Autodesk Fusion 360 part; units mm, degrees
(part 2 of 3)
sketch "Skizze16" plane through (0, 0, 3) normal (0, 0, -1) x (1, 0, 0)
  circle A0 centre (16.9122, 11.6198) radius 1
  circle A1 centre (77.0127, 20.2056) radius 2.5
  line L0 (81.1827, 15.7656) -> (79.9827, 16.6656)
  arc A2 (81.2427, 18.3456) -> (79.9827, 16.6656) centre (80.6127, 17.5056) ccw
  line L1 (81.2427, 18.3456) -> (82.4427, 17.4456)
  arc A3 (81.1827, 15.7656) -> (82.4427, 17.4456) centre (81.8127, 16.6056) ccw
  line L2 (72.7827, 22.0656) -> (71.5827, 22.9656)
  arc A4 (72.8427, 24.6456) -> (71.5827, 22.9656) centre (72.2127, 23.8056) ccw
  line L3 (72.8427, 24.6456) -> (74.0427, 23.7456)
  arc A5 (72.7827, 22.0656) -> (74.0427, 23.7456) centre (73.4127, 22.9056) ccw
  line L4 (72.5727, 16.0356) -> (73.4727, 17.2356)
  arc A6 (75.1527, 15.9756) -> (73.4727, 17.2356) centre (74.3127, 16.6056) ccw
  line L5 (75.1527, 15.9756) -> (74.2527, 14.7756)
  arc A7 (72.5727, 16.0356) -> (74.2527, 14.7756) centre (73.4127, 15.4056) ccw
  arc A8 (82.9846, 19.6249) -> (82.5459, 22.526) centre (77.0127, 20.2056) ccw
  arc A9 (83.8074, 23.8534) -> (82.5459, 22.526) centre (83.4681, 22.9127) ccw
  line L6 (83.8074, 23.8534) -> (87.1568, 22.6453)
  arc A10 (87.4261, 20.9112) -> (87.1568, 22.6453) centre (86.8175, 21.7046) ccw
  line L7 (87.4261, 20.9112) -> (84.5885, 18.7346)
  arc A11 (82.9846, 19.6249) -> (84.5885, 18.7346) centre (83.9799, 19.5281) ccw
  arc A12 (81.4527, 24.3756) -> (79.7727, 25.6356) centre (80.6127, 25.0056) ccw
  line L8 (81.4527, 24.3756) -> (80.5527, 23.1756)
  arc A13 (78.8727, 24.4356) -> (80.5527, 23.1756) centre (79.7127, 23.8056) ccw
  line L9 (78.8727, 24.4356) -> (79.7727, 25.6356)
  circle A14 centre (7.0127, 10.2056) radius 1
  line L10 (60.0865, 20.8143) -> (43.481, 18.4383)
  arc A15 (25.7008, 16.7003) -> (43.481, 18.4383) centre (15.1527, 216.4219) ccw
  line L11 (25.7008, 16.7003) -> (-2.9873, 15.1851)
  line L12 (-2.9873, 15.1851) -> (-2.9873, 11.7056)
  line L13 (-2.9873, 11.7056) -> (2.0127, 11.7056)
  arc A16 (2.0127, 8.7056) -> (2.0127, 11.7056) centre (2.0127, 10.2056) ccw
  line L14 (2.0127, 8.7056) -> (-2.9873, 8.7056)
  line L15 (-2.9873, 8.7056) -> (-2.9873, 5.7056)
  line L16 (-2.9873, 5.7056) -> (9.5815, 5.7056)
  arc A17 (9.5815, 5.7056) -> (14.161, 6.237) centre (9.5815, 25.7056) ccw
  line L17 (14.161, 6.237) -> (31.1237, 10.2271)
  arc A18 (39.9015, 11.8821) -> (31.1237, 10.2271) centre (54.0216, -87.116) ccw
  line L18 (39.9015, 11.8821) -> (60.934, 14.8819)
  arc A19 (72.34, 13.1475) -> (60.934, 14.8819) centre (63.758, -4.9177) ccw
  arc A20 (72.34, 13.1475) -> (74.5856, 13.1978) centre (73.4127, 15.4056) ccw
  arc A21 (77.8619, 14.266) -> (74.5856, 13.1978) centre (79.2772, 4.3667) ccw
  arc A22 (81.3049, 14.1577) -> (77.8619, 14.266) centre (79.2738, 4.3662) ccw
  arc A23 (81.3049, 14.1577) -> (83.2245, 14.5424) centre (81.8127, 16.6056) ccw
  line L19 (83.2245, 14.5424) -> (91.9997, 20.5467)
  arc A24 (91.9997, 20.5467) -> (91.4886, 24.0993) centre (90.8703, 22.1973) ccw
  line L20 (91.4886, 24.0993) -> (81.3855, 27.3832)
  arc A25 (81.3855, 27.3832) -> (79.4398, 27.2134) centre (80.6127, 25.0056) ccw
  arc A26 (76.1636, 26.1452) -> (79.4398, 27.2134) centre (74.7483, 36.0446) ccw
  arc A27 (72.7205, 26.2535) -> (76.1636, 26.1452) centre (74.7517, 36.045) ccw
  arc A28 (72.7205, 26.2535) -> (70.5506, 25.6731) centre (72.2127, 23.8056) ccw
  arc A29 (60.0865, 20.8143) -> (70.5506, 25.6731) centre (57.2537, 40.6127) ccw
  circle A30 centre (16.9122, 11.6198) radius 1.5
  circle A31 centre (7.0127, 10.2056) radius 1.5
  dimension "d177" = 3
  dimension "d178" = 3
  constraint concentric A0 A30
  constraint concentric A14 A31
  measures "d177" diameter of A30
  measures "d178" diameter of A31
extrude "Extrusion1'''" cut sketch "Skizze16" against normal blind 3 contours A30 | A31 sketch seen with x (-0.6, -0.8, 0) y (0.8, -0.6, 0) z (0, 0, 1) at (-23.2665, 43.7378, -3) bodies 10 in component "Component''"
sketch "Skizze17" plane through (0, 0, 3) normal (0, 0, -1) x (1, 0, 0)
  circle A0 centre (-22.8868, 11.6198) radius 1
  circle A1 centre (-82.9873, 20.2056) radius 2.5
  line L0 (-85.9573, 16.6656) -> (-87.1573, 15.7656)
  arc A2 (-88.4173, 17.4456) -> (-87.1573, 15.7656) centre (-87.7873, 16.6056) ccw
  line L1 (-88.4173, 17.4456) -> (-87.2173, 18.3456)
  arc A3 (-85.9573, 16.6656) -> (-87.2173, 18.3456) centre (-86.5873, 17.5056) ccw
  line L2 (-77.5573, 22.9656) -> (-78.7573, 22.0656)
  arc A4 (-80.0173, 23.7456) -> (-78.7573, 22.0656) centre (-79.3873, 22.9056) ccw
  line L3 (-80.0173, 23.7456) -> (-78.8173, 24.6456)
  arc A5 (-77.5573, 22.9656) -> (-78.8173, 24.6456) centre (-78.1873, 23.8056) ccw
  line L4 (-79.4473, 17.2356) -> (-78.5473, 16.0356)
  arc A6 (-80.2273, 14.7756) -> (-78.5473, 16.0356) centre (-79.3873, 15.4056) ccw
  line L5 (-80.2273, 14.7756) -> (-81.1273, 15.9756)
  arc A7 (-79.4473, 17.2356) -> (-81.1273, 15.9756) centre (-80.2873, 16.6056) ccw
  arc A8 (-88.5204, 22.526) -> (-88.9591, 19.6249) centre (-82.9873, 20.2056) ccw
  arc A9 (-90.563, 18.7346) -> (-88.9591, 19.6249) centre (-89.9544, 19.5281) ccw
  line L6 (-90.563, 18.7346) -> (-93.4007, 20.9112)
  arc A10 (-93.1314, 22.6453) -> (-93.4007, 20.9112) centre (-92.7921, 21.7046) ccw
  line L7 (-93.1314, 22.6453) -> (-89.7819, 23.8534)
  arc A11 (-88.5204, 22.526) -> (-89.7819, 23.8534) centre (-89.4426, 22.9127) ccw
  arc A12 (-85.7473, 25.6356) -> (-87.4273, 24.3756) centre (-86.5873, 25.0056) ccw
  line L8 (-85.7473, 25.6356) -> (-84.8473, 24.4356)
  arc A13 (-86.5273, 23.1756) -> (-84.8473, 24.4356) centre (-85.6873, 23.8056) ccw
  line L9 (-86.5273, 23.1756) -> (-87.4273, 24.3756)
  circle A14 centre (-12.9873, 10.2056) radius 1
  line L10 (-49.4555, 18.4383) -> (-66.061, 20.8143)
  arc A15 (-76.5252, 25.6731) -> (-66.061, 20.8143) centre (-63.2282, 40.6127) ccw
  arc A16 (-76.5252, 25.6731) -> (-78.6951, 26.2535) centre (-78.1873, 23.8056) ccw
  arc A17 (-82.1381, 26.1452) -> (-78.6951, 26.2535) centre (-80.7262, 36.045) ccw
  arc A18 (-85.4144, 27.2134) -> (-82.1381, 26.1452) centre (-80.7228, 36.0446) ccw
  arc A19 (-85.4144, 27.2134) -> (-87.3601, 27.3832) centre (-86.5873, 25.0056) ccw
  line L11 (-87.3601, 27.3832) -> (-97.4631, 24.0993)
  arc A20 (-97.4631, 24.0993) -> (-97.9743, 20.5467) centre (-96.8449, 22.1973) ccw
  line L12 (-97.9743, 20.5467) -> (-89.199, 14.5424)
  arc A21 (-89.199, 14.5424) -> (-87.2795, 14.1577) centre (-87.7873, 16.6056) ccw
  arc A22 (-83.8364, 14.266) -> (-87.2795, 14.1577) centre (-85.2483, 4.3662) ccw
  arc A23 (-80.5602, 13.1978) -> (-83.8364, 14.266) centre (-85.2517, 4.3667) ccw
  arc A24 (-80.5602, 13.1978) -> (-78.3145, 13.1475) centre (-79.3873, 15.4056) ccw
  arc A25 (-66.9085, 14.8819) -> (-78.3145, 13.1475) centre (-69.7326, -4.9177) ccw
  line L13 (-66.9085, 14.8819) -> (-45.8761, 11.8821)
  arc A26 (-37.0983, 10.2271) -> (-45.8761, 11.8821) centre (-59.9962, -87.116) ccw
  line L14 (-37.0983, 10.2271) -> (-20.1356, 6.237)
  arc A27 (-20.1356, 6.237) -> (-15.556, 5.7056) centre (-15.556, 25.7056) ccw
  line L15 (-15.556, 5.7056) -> (-2.9873, 5.7056)
  line L16 (-2.9873, 5.7056) -> (-2.9873, 8.7056)
  line L17 (-2.9873, 8.7056) -> (-7.9873, 8.7056)
  arc A28 (-7.9873, 11.7056) -> (-7.9873, 8.7056) centre (-7.9873, 10.2056) ccw
  line L18 (-7.9873, 11.7056) -> (-2.9873, 11.7056)
  line L19 (-2.9873, 11.7056) -> (-2.9873, 15.1851)
  line L20 (-2.9873, 15.1851) -> (-31.6754, 16.7003)
  arc A29 (-49.4555, 18.4383) -> (-31.6754, 16.7003) centre (-21.1273, 216.4219) ccw
  circle A30 centre (-22.8868, 11.6198) radius 1.5
  circle A31 centre (-12.9873, 10.2056) radius 1.5
  dimension "d181" = 3
  dimension "d182" = 3
  constraint concentric A0 A30
  constraint concentric A14 A31
  measures "d181" diameter of A30
  measures "d182" diameter of A31
extrude "Extrusion1''''" cut sketch "Skizze17" against normal blind 3 contours A30 | A31 sketch seen with x (0.6, 0.8, 0) y (0.8, -0.6, 0) z (0, 0, -1) at (-18.7221, 22.2947, 6) bodies 11 in component "Component'''"
sketch "Skizze18" plane through (0, 0, 3) normal (0, 0, -1) x (1, 0, 0)
  circle A0 centre (-20.7786, -30.2009) radius 1
  arc A1 (-65.0305, -85.2371) -> (-65.3296, -83.1585) centre (-65.18, -84.1978) ccw
  line L0 (-65.0305, -85.2371) -> (-66.5152, -85.4508)
  arc A2 (-66.8143, -83.3722) -> (-66.5152, -85.4508) centre (-66.6647, -84.4115) ccw
  line L1 (-66.8143, -83.3722) -> (-65.3296, -83.1585)
  arc A3 (-65.3866, -87.3355) -> (-67.1533, -87.8235) centre (-66.1634, -87.9652) ccw
  arc A4 (-65.3866, -87.3355) -> (-63.0387, -89.0932) centre (-60.7259, -83.5569) ccw
  arc A5 (-63.0094, -90.9259) -> (-63.0387, -89.0932) centre (-63.4241, -90.016) ccw
  line L2 (-63.0094, -90.9259) -> (-66.2541, -92.4046)
  arc A6 (-67.6587, -91.3529) -> (-66.2541, -92.4046) centre (-66.6688, -91.4947) ccw
  line L3 (-67.6587, -91.3529) -> (-67.1533, -87.8235)
  arc A7 (-60.5412, -77.4685) -> (-62.6198, -77.7676) centre (-61.5805, -77.6181) ccw
  line L4 (-60.5412, -77.4685) -> (-60.3275, -78.9532)
  arc A8 (-62.4061, -79.2523) -> (-60.3275, -78.9532) centre (-61.3668, -79.1028) ccw
  line L5 (-62.4061, -79.2523) -> (-62.6198, -77.7676)
  circle A9 centre (-60.7259, -83.5569) radius 2.5
  circle A10 centre (-12.9873, -19.7944) radius 1
  arc A11 (-59.0457, -87.8615) -> (-61.1243, -88.1606) centre (-60.085, -88.011) ccw
  line L6 (-59.0457, -87.8615) -> (-58.832, -89.3462)
  arc A12 (-60.9106, -89.6453) -> (-58.832, -89.3462) centre (-59.8713, -89.4957) ccw
  line L7 (-60.9106, -89.6453) -> (-61.1243, -88.1606)
  line L8 (-56.4213, -81.8767) -> (-54.9366, -81.663)
  arc A13 (-54.6375, -83.7416) -> (-54.9366, -81.663) centre (-54.7871, -82.7023) ccw
  line L9 (-54.6375, -83.7416) -> (-56.1222, -83.9553)
  arc A14 (-56.4213, -81.8767) -> (-56.1222, -83.9553) centre (-56.2718, -82.916) ccw
  arc A15 (-68.3484, -81.9285) -> (-69.636, -83.9975) centre (-66.6647, -84.4115) ccw
  line L10 (-69.636, -83.9975) -> (-71.0974, -94.488)
  arc A16 (-71.0974, -94.488) -> (-68.294, -96.587) centre (-69.1165, -94.7639) ccw
  line L11 (-68.294, -96.587) -> (-58.6376, -92.2303)
  arc A17 (-58.6376, -92.2303) -> (-57.0144, -90.411) centre (-59.8713, -89.4957) ccw
  arc A18 (-53.1034, -85.1853) -> (-57.0144, -90.411) centre (-47.4911, -93.4619) ccw
  arc A19 (-53.1034, -85.1853) -> (-51.788, -82.7784) centre (-54.7871, -82.7023) ccw
  arc A20 (-47.8066, -71.3016) -> (-51.788, -82.7784) centre (-31.7945, -83.2854) ccw
  line L12 (-47.8066, -71.3016) -> (-30.9597, -48.7917)
  arc A21 (-25.5822, -42.2094) -> (-30.9597, -48.7917) centre (49.1009, -108.7108) ccw
  line L13 (-25.5822, -42.2094) -> (-21.1501, -37.232)
  arc A22 (-21.1501, -37.232) -> (-16.2298, -30.7009) centre (-58.4917, -3.9813) ccw
  line L14 (-16.2298, -30.7009) -> (-13.6512, -26.6224)
  arc A23 (-9.4251, -24.2944) -> (-13.6512, -26.6224) centre (-9.4251, -29.2944) ccw
  line L15 (-9.4251, -24.2944) -> (-2.9873, -24.2944)
  line L16 (-2.9873, -24.2944) -> (-2.9873, -21.2944)
  line L17 (-2.9873, -21.2944) -> (-7.9873, -21.2944)
  arc A24 (-7.9873, -18.2944) -> (-7.9873, -21.2944) centre (-7.9873, -19.7944) ccw
  line L18 (-7.9873, -18.2944) -> (-2.9873, -18.2944)
  line L19 (-2.9873, -18.2944) -> (-2.9873, -15.2944)
  line L20 (-2.9873, -15.2944) -> (-13.8886, -15.2944)
  arc A25 (-13.8886, -15.2944) -> (-18.1306, -17.6477) centre (-13.8886, -20.2944) ccw
  line L21 (-18.1306, -17.6477) -> (-30.9484, -38.1918)
  arc A26 (-35.7499, -45.2053) -> (-30.9484, -38.1918) centre (-115.7896, 14.7418) ccw
  line L22 (-35.7499, -45.2053) -> (-52.6043, -67.7088)
  arc A27 (-62.4977, -74.7617) -> (-52.6043, -67.7088) centre (-68.6122, -55.7193) ccw
  arc A28 (-62.4977, -74.7617) -> (-64.4374, -76.7028) centre (-61.5805, -77.6181) ccw
  arc A29 (-68.3484, -81.9285) -> (-64.4374, -76.7028) centre (-73.9607, -73.6518) ccw
  circle A30 centre (-20.7786, -30.2009) radius 1.5
  circle A31 centre (-12.9873, -19.7944) radius 1.5
  dimension "d185" = 3
  dimension "d186" = 3
  constraint concentric A0 A30
  constraint concentric A10 A31
  measures "d185" diameter of A30
  measures "d186" diameter of A31
extrude "Extrusion1'''''" cut sketch "Skizze18" against normal blind 3 contours A30 | A31 sketch seen with x (0.989831, -0.142249, 0) y (-0.142249, -0.989831, 0) z (0, 0, -1) at (-24.4554, -5.7072, 6) bodies 12 in component "Component''''"
sketch "Skizze19" plane through (0, 0, 0) normal (0, 0, -1) x (1, 0, 0)
  circle A0 centre (-10.9873, -60.7944) radius 1
  circle A1 centre (7.0127, -49.2944) radius 1
  circle A2 centre (-10.9873, -12.7944) radius 1
  circle A3 centre (-22.8868, 11.6198) radius 1
  circle A4 centre (7.0127, -19.7944) radius 1
  circle A5 centre (7.0127, 10.2056) radius 1
  arc A6 (4.4716, -52.3625) -> (3.467, -47.3835) centre (-2.4249, -51.1632) ccw
  line L0 (4.4716, -52.3625) -> (3.9295, -55.4797)
  arc A7 (-0.0113, -58.7944) -> (3.9295, -55.4797) centre (-0.0113, -54.7944) ccw
  line L1 (-0.0113, -58.7944) -> (-5.9632, -58.7944)
  arc A8 (-9.904, -55.4797) -> (-5.9632, -58.7944) centre (-5.9632, -54.7944) ccw
  line L2 (-9.904, -55.4797) -> (-10.4462, -52.3625)
  arc A9 (-9.4415, -47.3835) -> (-10.4462, -52.3625) centre (-3.5497, -51.1632) ccw
  line L3 (-9.4415, -47.3835) -> (-4.0198, -38.932)
  arc A10 (-3.1781, -38.4719) -> (-4.0198, -38.932) centre (-3.1781, -39.4719) ccw
  line L4 (-3.1781, -38.4719) -> (-2.7964, -38.4719)
  arc A11 (-1.9547, -38.932) -> (-2.7964, -38.4719) centre (-2.7964, -39.4719) ccw
  line L5 (-1.9547, -38.932) -> (3.467, -47.3835)
  arc A12 (-10.6956, -31.3597) -> (-10.9873, -32.7585) centre (-7.4873, -32.7585) ccw
  arc A13 (-10.6956, -31.3597) -> (-10.4873, -30.3606) centre (-12.9873, -30.3606) ccw
  line L6 (-10.4873, -30.3606) -> (-10.4873, -28.821)
  arc A14 (-8.6429, -28.2852) -> (-10.4873, -28.821) centre (-9.4873, -28.821) ccw
  line L7 (-8.6429, -28.2852) -> (-6.2521, -32.0531)
  arc A15 (-5.9408, -33.1247) -> (-6.2521, -32.0531) centre (-7.9408, -33.1247) ccw
  line L8 (-5.9408, -33.1247) -> (-5.9408, -35.784)
  arc A16 (-6.2574, -36.8639) -> (-5.9408, -35.784) centre (-7.9408, -35.784) ccw
  line L9 (-6.2574, -36.8639) -> (-9.1456, -41.3661)
  arc A17 (-10.9873, -40.8261) -> (-9.1456, -41.3661) centre (-9.9873, -40.8261) ccw
  line L10 (-10.9873, -40.8261) -> (-10.9873, -32.7585)
  circle A18 centre (5.0127, -12.7944) radius 1
  arc A19 (-2.8219, -30.4719) -> (-1.9776, -30.0077) centre (-2.8219, -29.4719) ccw
  line L11 (-2.8219, -30.4719) -> (-3.1526, -30.4719)
  arc A20 (-3.997, -30.0077) -> (-3.1526, -30.4719) centre (-3.1526, -29.4719) ccw
  line L12 (-3.997, -30.0077) -> (-6.6478, -25.8302)
  arc A21 (-5.8034, -24.2944) -> (-6.6478, -25.8302) centre (-5.8034, -25.2944) ccw
  line L13 (-5.8034, -24.2944) -> (-0.1711, -24.2944)
  arc A22 (0.6732, -25.8302) -> (-0.1711, -24.2944) centre (-0.1711, -25.2944) ccw
  line L14 (0.6732, -25.8302) -> (-1.9776, -30.0077)
  line L15 (2.0127, 8.7056) -> (-7.9873, 8.7056)
  arc A23 (-7.9873, 11.7056) -> (-7.9873, 8.7056) centre (-7.9873, 10.2056) ccw
  line L16 (-7.9873, 11.7056) -> (2.0127, 11.7056)
  arc A24 (2.0127, 8.7056) -> (2.0127, 11.7056) centre (2.0127, 10.2056) ccw
  circle A25 centre (16.9122, 11.6198) radius 1
  circle A26 centre (14.804, -30.2009) radius 1
  circle A27 centre (-12.9873, 10.2056) radius 1
  circle A28 centre (-12.9873, -19.7944) radius 1
  circle A29 centre (5.0127, 3.2056) radius 1
  line L17 (2.0127, -21.2944) -> (-7.9873, -21.2944)
  arc A30 (-7.9873, -18.2944) -> (-7.9873, -21.2944) centre (-7.9873, -19.7944) ccw
  line L18 (-7.9873, -18.2944) -> (2.0127, -18.2944)
  arc A31 (2.0127, -21.2944) -> (2.0127, -18.2944) centre (2.0127, -19.7944) ccw
  circle A32 centre (5.0127, -60.7944) radius 1
  circle A33 centre (-12.9873, -49.2944) radius 1
  circle A34 centre (-10.9873, 3.2056) radius 1
  circle A35 centre (-20.7786, -30.2009) radius 1
  line L19 (3.5127, -1.2944) -> (3.5127, -8.2944)
  arc A36 (0.5127, -11.2944) -> (3.5127, -8.2944) centre (0.5127, -8.2944) ccw
  line L20 (0.5127, -11.2944) -> (-6.4873, -11.2944)
  arc A37 (-9.4873, -8.2944) -> (-6.4873, -11.2944) centre (-6.4873, -8.2944) ccw
  line L21 (-9.4873, -8.2944) -> (-9.4873, -1.2944)
  arc A38 (-6.4873, 1.7056) -> (-9.4873, -1.2944) centre (-6.4873, -1.2944) ccw
  line L22 (-6.4873, 1.7056) -> (0.5127, 1.7056)
  arc A39 (3.5127, -1.2944) -> (0.5127, 1.7056) centre (0.5127, -1.2944) ccw
  arc A40 (4.5127, -28.821) -> (2.6684, -28.2852) centre (3.5127, -28.821) ccw
  line L23 (4.5127, -28.821) -> (4.5127, -30.3606)
  arc A41 (4.5127, -30.3606) -> (4.7211, -31.3597) centre (7.0127, -30.3606) ccw
  arc A42 (5.0127, -32.7585) -> (4.7211, -31.3597) centre (1.5127, -32.7585) ccw
  line L24 (5.0127, -32.7585) -> (5.0127, -40.8261)
  arc A43 (3.171, -41.3661) -> (5.0127, -40.8261) centre (4.0127, -40.8261) ccw
  line L25 (3.171, -41.3661) -> (0.2829, -36.8639)
  arc A44 (-0.0338, -35.784) -> (0.2829, -36.8639) centre (1.9662, -35.784) ccw
  line L26 (-0.0338, -35.784) -> (-0.0338, -33.1247)
  arc A45 (0.2775, -32.0531) -> (-0.0338, -33.1247) centre (1.9662, -33.1247) ccw
  line L27 (0.2775, -32.0531) -> (2.6684, -28.2852)
  circle A46 centre (-12.9873, -29.2944) radius 1
  circle A47 centre (7.0127, -29.2944) radius 1
  arc A48 (8.5127, -45.5527) -> (9.1794, -48.0472) centre (13.5127, -45.5527) ccw
  line L28 (8.5127, -45.5527) -> (8.5127, -33.6896)
  arc A49 (11.133, -32.6921) -> (8.5127, -33.6896) centre (10.0127, -33.6896) ccw
  line L29 (11.133, -32.6921) -> (11.5192, -33.1258)
  arc A50 (11.5192, -33.1258) -> (18.5356, -27.8727) centre (14.804, -30.2009) ccw
  line L30 (18.5356, -27.8727) -> (12.3422, -17.946)
  arc A51 (10.8263, -12.6526) -> (12.3422, -17.946) centre (20.8263, -12.6526) ccw
  line L31 (10.8263, -12.6526) -> (10.8263, 1.4922)
  arc A52 (14.6814, 6.3594) -> (10.8263, 1.4922) centre (15.8263, 1.4922) ccw
  line L32 (14.6814, 6.3594) -> (17.9678, 7.1324)
  arc A53 (17.9678, 7.1324) -> (16.6691, 16.2233) centre (16.9122, 11.6198) ccw
  line L33 (16.6691, 16.2233) -> (-0.3502, 15.3244)
  arc A54 (-5.6243, 15.3244) -> (-0.3502, 15.3244) centre (-2.9873, 65.2548) ccw
  line L34 (-5.6243, 15.3244) -> (-22.6436, 16.2233)
  arc A55 (-22.6436, 16.2233) -> (-23.9423, 7.1324) centre (-22.8868, 11.6198) ccw
  line L35 (-23.9423, 7.1324) -> (-20.6559, 6.3594)
  arc A56 (-16.8008, 1.4922) -> (-20.6559, 6.3594) centre (-21.8008, 1.4922) ccw
  line L36 (-16.8008, 1.4922) -> (-16.8008, -12.6526)
  arc A57 (-18.3167, -17.946) -> (-16.8008, -12.6526) centre (-26.8008, -12.6526) ccw
  line L37 (-18.3167, -17.946) -> (-24.5102, -27.8727)
  arc A58 (-24.5102, -27.8727) -> (-17.4938, -33.1258) centre (-20.7786, -30.2009) ccw
  line L38 (-17.4938, -33.1258) -> (-17.1075, -32.6921)
  arc A59 (-14.4873, -33.6896) -> (-17.1075, -32.6921) centre (-15.9873, -33.6896) ccw
  line L39 (-14.4873, -33.6896) -> (-14.4873, -45.5527)
  arc A60 (-15.1539, -48.0472) -> (-14.4873, -45.5527) centre (-19.4873, -45.5527) ccw
  arc A61 (-15.1539, -48.0472) -> (-14.9651, -50.8235) centre (-12.9873, -49.2944) ccw
  arc A62 (-14.0092, -52.946) -> (-14.9651, -50.8235) centre (-18.9209, -53.8816) ccw
  line L40 (-14.0092, -52.946) -> (-13.1609, -57.3995)
  arc A63 (-13.349, -59.9746) -> (-13.1609, -57.3995) centre (-18.0726, -58.335) ccw
  arc A64 (-13.349, -59.9746) -> (-10.0897, -63.1277) centre (-10.9873, -60.7944) ccw
  arc A65 (-8.2947, -62.7944) -> (-10.0897, -63.1277) centre (-8.2947, -67.7944) ccw
  line L41 (-8.2947, -62.7944) -> (2.3201, -62.7944)
  arc A66 (4.1152, -63.1277) -> (2.3201, -62.7944) centre (2.3201, -67.7944) ccw
  arc A67 (4.1152, -63.1277) -> (7.3745, -59.9746) centre (5.0127, -60.7944) ccw
  arc A68 (7.1863, -57.3995) -> (7.3745, -59.9746) centre (12.098, -58.335) ccw
  line L42 (7.1863, -57.3995) -> (8.0346, -52.946)
  arc A69 (8.9906, -50.8235) -> (8.0346, -52.946) centre (12.9463, -53.8816) ccw
  arc A70 (8.9906, -50.8235) -> (9.1794, -48.0472) centre (7.0127, -49.2944) ccw
  circle A71 centre (-22.8868, 11.6198) radius 1.5
  circle A72 centre (-12.9873, 10.2056) radius 1.5
  circle A73 centre (7.0127, 10.2056) radius 1.5
  circle A74 centre (16.9122, 11.6198) radius 1.5
  circle A75 centre (7.0127, -19.7944) radius 1.5
  circle A76 centre (-12.9873, -19.7944) radius 1.5
  circle A77 centre (-20.7786, -30.2009) radius 1.5
  circle A78 centre (-12.9873, -29.2944) radius 1.5
  circle A79 centre (7.0127, -29.2944) radius 1.5
  circle A80 centre (14.804, -30.2009) radius 1.5
  circle A81 centre (-12.9873, -49.2944) radius 1.5
  circle A82 centre (-10.9873, -60.7944) radius 1.5
  circle A83 centre (5.0127, -60.7944) radius 1.5
  circle A84 centre (7.0127, -49.2944) radius 1.5
  circle A85 centre (5.0127, -60.7944) radius 3.5
  circle A86 centre (-10.9873, -60.7944) radius 3.5
  circle A87 centre (-12.9873, -49.2944) radius 3.5
  circle A88 centre (7.0127, -49.2944) radius 3.5
  circle A89 centre (-12.9873, -29.2944) radius 3.5
  circle A90 centre (7.0127, -29.2944) radius 3.5
  circle A91 centre (-10.9873, 3.2056) radius 1.5
  circle A92 centre (-10.9873, -12.7944) radius 1.5
  circle A93 centre (5.0127, -12.7944) radius 1.5
  circle A94 centre (5.0127, 3.2056) radius 1.5
  dimension "d189" = 3
  dimension "d190" = 3
  dimension "d191" = 3
  dimension "d192" = 3
  dimension "d193" = 3
  dimension "d194" = 3
  dimension "d195" = 3
  dimension "d196" = 3
  dimension "d197" = 3
  dimension "d198" = 3
  dimension "d199" = 3
  dimension "d200" = 3
  dimension "d201" = 3
  dimension "d202" = 3
  dimension "d203" = 7
  dimension "d204" = 7
  dimension "d205" = 7
  dimension "d206" = 7
  dimension "d207" = 7
  dimension "d208" = 7
  dimension "d235" = 3
  dimension "d236" = 3
  dimension "d237" = 3
  dimension "d238" = 3
  constraint concentric A3 A71
  constraint concentric A27 A72
  constraint concentric A5 A73
  constraint concentric A25 A74
  constraint concentric A4 A75
  constraint concentric A28 A76
  constraint concentric A35 A77
  constraint concentric A46 A78
  constraint concentric A47 A79
  constraint concentric A26 A80
  constraint concentric A33 A81
  constraint concentric A0 A82
  constraint concentric A32 A83
  constraint concentric A1 A84
  constraint concentric A83 A85
  constraint concentric A82 A86
  constraint concentric A33 A87
  constraint concentric A84 A88
  constraint concentric A78 A89
  constraint concentric A79 A90
  constraint concentric A34 A91
  constraint concentric A2 A92
  constraint concentric A18 A93
  constraint concentric A29 A94
  measures "d189" diameter of A71
  measures "d190" diameter of A72
  measures "d191" diameter of A73
  measures "d192" diameter of A74
  measures "d193" diameter of A75
  measures "d194" diameter of A76
  measures "d195" diameter of A77
  measures "d196" diameter of A78
  measures "d197" diameter of A79
  measures "d198" diameter of A80
  measures "d199" diameter of A81
  measures "d200" diameter of A82
  measures "d201" diameter of A83
  measures "d202" diameter of A84
  measures "d203" diameter of A85
  measures "d204" diameter of A86
  measures "d205" diameter of A87
  measures "d206" diameter of A88
  measures "d207" diameter of A89
  measures "d208" diameter of A90
  measures "d235" diameter of A91
  measures "d236" diameter of A92
  measures "d237" diameter of A93
  measures "d238" diameter of A94
extrude "Extrusion1''''''" cut sketch "Skizze19" against normal blind 3 contours A71 | A72 | A73 | A74 | A75 | A76 | A77 | A80 | A82 | A83 | A91 | A92 | A93 | A94 sketch seen with x (1, 0, 0) y (0, 1, 0) z (0, 0, 1) at (2.9873, 0.2056, 0) bodies 13 in component "Component'''''"
extrude "Extrusion2'''" add sketch "Skizze19" against normal blind 3 contours L41 A66 A67 A68 A85 | A63 A64 A65 L41 A86 picked at (7.6038, -59.5802) picked at (-13.5291, -59.4774) sketch seen with x (1, 0, 0) y (0, 1, 0) z (0, 0, 1) at (2.9873, 0.2056, 0) bodies 13 in component "Component'''''"
fillet "Abrundung1''" radius 5 4 edges at (-10.0971, 58.1978, 1.5) (-5.1277, 63, 1.5) (5.1277, 63, 1.5) (10.0971, 58.1978, 1.5) on bodies 13 in component "Component'''''"
sketch "Skizze20" plane through (0, 0, 3) normal (0, 0, 1) x (-1, 0, 0)
  circle A0 centre (12.9873, 10.2056) radius 1.5
  circle A1 centre (-14.804, -30.2009) radius 1.5
  circle A2 centre (10.9873, -60.7944) radius 1.5
  circle A3 centre (20.7786, -30.2009) radius 1.5
  circle A4 centre (-5.0127, -60.7944) radius 1.5
  circle A5 centre (-7.0127, -19.7944) radius 1.5
  circle A6 centre (-7.0127, 10.2056) radius 1.5
  circle A7 centre (22.8868, 11.6198) radius 1.5
  circle A8 centre (12.9873, -19.7944) radius 1.5
  circle A9 centre (-16.9122, 11.6198) radius 1.5
  line L0 (-3.467, -47.3835) -> (1.9547, -38.932)
  arc A10 (2.7964, -38.4719) -> (1.9547, -38.932) centre (2.7964, -39.4719) ccw
  line L1 (2.7964, -38.4719) -> (3.1781, -38.4719)
  arc A11 (4.0198, -38.932) -> (3.1781, -38.4719) centre (3.1781, -39.4719) ccw
  line L2 (4.0198, -38.932) -> (9.4415, -47.3835)
  line L3 (10.4462, -52.3625) -> (9.904, -55.4797)
  arc A12 (5.9632, -58.7944) -> (9.904, -55.4797) centre (5.9632, -54.7944) ccw
  line L4 (5.9632, -58.7944) -> (0.0113, -58.7944)
  arc A13 (-3.9295, -55.4797) -> (0.0113, -58.7944) centre (0.0113, -54.7944) ccw
  line L5 (-3.9295, -55.4797) -> (-4.4716, -52.3625)
  line L6 (10.9873, -32.7585) -> (10.9873, -40.8261)
  arc A14 (9.1456, -41.3661) -> (10.9873, -40.8261) centre (9.9873, -40.8261) ccw
  line L7 (9.1456, -41.3661) -> (6.2574, -36.8639)
  arc A15 (5.9408, -35.784) -> (6.2574, -36.8639) centre (7.9408, -35.784) ccw
  line L8 (5.9408, -35.784) -> (5.9408, -33.1247)
  arc A16 (6.2521, -32.0531) -> (5.9408, -33.1247) centre (7.9408, -33.1247) ccw
  line L9 (6.2521, -32.0531) -> (8.6429, -28.2852)
  arc A17 (1.9776, -30.0077) -> (2.8219, -30.4719) centre (2.8219, -29.4719) ccw
  line L10 (1.9776, -30.0077) -> (-0.6732, -25.8302)
  arc A18 (0.1711, -24.2944) -> (-0.6732, -25.8302) centre (0.1711, -25.2944) ccw
  line L11 (0.1711, -24.2944) -> (5.8034, -24.2944)
  arc A19 (6.6478, -25.8302) -> (5.8034, -24.2944) centre (5.8034, -25.2944) ccw
  line L12 (6.6478, -25.8302) -> (3.997, -30.0077)
  arc A20 (3.1526, -30.4719) -> (3.997, -30.0077) centre (3.1526, -29.4719) ccw
  line L13 (3.1526, -30.4719) -> (2.8219, -30.4719)
  line L14 (7.9873, 8.7056) -> (-2.0127, 8.7056)
  arc A21 (-2.0127, 11.7056) -> (-2.0127, 8.7056) centre (-2.0127, 10.2056) ccw
  line L15 (-2.0127, 11.7056) -> (7.9873, 11.7056)
  arc A22 (7.9873, 8.7056) -> (7.9873, 11.7056) centre (7.9873, 10.2056) ccw
  line L16 (7.9873, -21.2944) -> (-2.0127, -21.2944)
  arc A23 (-2.0127, -18.2944) -> (-2.0127, -21.2944) centre (-2.0127, -19.7944) ccw
  line L17 (-2.0127, -18.2944) -> (7.9873, -18.2944)
  arc A24 (7.9873, -21.2944) -> (7.9873, -18.2944) centre (7.9873, -19.7944) ccw
  line L18 (-3.5127, -8.2944) -> (-3.5127, -1.2944)
  arc A25 (-0.5127, 1.7056) -> (-3.5127, -1.2944) centre (-0.5127, -1.2944) ccw
  line L19 (-0.5127, 1.7056) -> (6.4873, 1.7056)
  arc A26 (9.4873, -1.2944) -> (6.4873, 1.7056) centre (6.4873, -1.2944) ccw
  line L20 (9.4873, -1.2944) -> (9.4873, -8.2944)
  arc A27 (6.4873, -11.2944) -> (9.4873, -8.2944) centre (6.4873, -8.2944) ccw
  line L21 (6.4873, -11.2944) -> (-0.5127, -11.2944)
  arc A28 (-3.5127, -8.2944) -> (-0.5127, -11.2944) centre (-0.5127, -8.2944) ccw
  line L22 (-2.6684, -28.2852) -> (-0.2775, -32.0531)
  arc A29 (0.0338, -33.1247) -> (-0.2775, -32.0531) centre (-1.9662, -33.1247) ccw
  line L23 (0.0338, -33.1247) -> (0.0338, -35.784)
  arc A30 (-0.2829, -36.8639) -> (0.0338, -35.784) centre (-1.9662, -35.784) ccw
  line L24 (-0.2829, -36.8639) -> (-3.171, -41.3661)
  arc A31 (-5.0127, -40.8261) -> (-3.171, -41.3661) centre (-4.0127, -40.8261) ccw
  line L25 (-5.0127, -40.8261) -> (-5.0127, -32.7585)
  line L26 (-8.0346, -52.946) -> (-7.5111, -55.6946)
  arc A32 (-8.0639, -59.0797) -> (-7.5111, -55.6946) centre (-12.4228, -56.6301) ccw
  arc A33 (-8.0639, -59.0797) -> (-3.0273, -63.6767) centre (-5.0127, -60.7944) ccw
  arc A34 (-0.1909, -62.7944) -> (-3.0273, -63.6767) centre (-0.1909, -67.7944) ccw
  line L27 (-0.1909, -62.7944) -> (6.1654, -62.7944)
  arc A35 (9.0018, -63.6767) -> (6.1654, -62.7944) centre (6.1654, -67.7944) ccw
  arc A36 (9.0018, -63.6767) -> (14.0385, -59.0797) centre (10.9873, -60.7944) ccw
  arc A37 (13.4856, -55.6946) -> (14.0385, -59.0797) centre (18.3973, -56.6301) ccw
  line L28 (13.4856, -55.6946) -> (14.0092, -52.946)
  line L29 (14.4873, -45.5527) -> (14.4873, -33.6896)
  arc A38 (17.1075, -32.6921) -> (14.4873, -33.6896) centre (15.9873, -33.6896) ccw
  line L30 (17.1075, -32.6921) -> (17.4938, -33.1258)
  arc A39 (17.4938, -33.1258) -> (24.5102, -27.8727) centre (20.7786, -30.2009) ccw
  line L31 (24.5102, -27.8727) -> (18.3167, -17.946)
  arc A40 (16.8008, -12.6526) -> (18.3167, -17.946) centre (26.8008, -12.6526) ccw
  line L32 (16.8008, -12.6526) -> (16.8008, 1.4922)
  arc A41 (20.6559, 6.3594) -> (16.8008, 1.4922) centre (21.8008, 1.4922) ccw
  line L33 (20.6559, 6.3594) -> (23.9423, 7.1324)
  arc A42 (23.9423, 7.1324) -> (22.6436, 16.2233) centre (22.8868, 11.6198) ccw
  line L34 (22.6436, 16.2233) -> (5.6243, 15.3244)
  arc A43 (0.3502, 15.3244) -> (5.6243, 15.3244) centre (2.9873, 65.2548) ccw
  line L35 (0.3502, 15.3244) -> (-16.6691, 16.2233)
  arc A44 (-16.6691, 16.2233) -> (-17.9678, 7.1324) centre (-16.9122, 11.6198) ccw
  line L36 (-17.9678, 7.1324) -> (-14.6814, 6.3594)
  arc A45 (-10.8263, 1.4922) -> (-14.6814, 6.3594) centre (-15.8263, 1.4922) ccw
  line L37 (-10.8263, 1.4922) -> (-10.8263, -12.6526)
  arc A46 (-12.3422, -17.946) -> (-10.8263, -12.6526) centre (-20.8263, -12.6526) ccw
  line L38 (-12.3422, -17.946) -> (-18.5356, -27.8727)
  arc A47 (-18.5356, -27.8727) -> (-11.5192, -33.1258) centre (-14.804, -30.2009) ccw
  line L39 (-11.5192, -33.1258) -> (-11.133, -32.6921)
  arc A48 (-8.5127, -33.6896) -> (-11.133, -32.6921) centre (-10.0127, -33.6896) ccw
  line L40 (-8.5127, -33.6896) -> (-8.5127, -45.5527)
  circle A49 centre (12.9873, -29.2944) radius 2
  circle A50 centre (-7.0127, -29.2944) radius 2
  circle A51 centre (-7.0127, -49.2944) radius 1
  circle A52 centre (12.9873, -49.2944) radius 1
  circle A53 centre (12.9873, -29.2944) radius 1
  circle A54 centre (-7.0127, -29.2944) radius 1
  arc A55 (-3.467, -47.3835) -> (-4.4716, -52.3625) centre (2.4249, -51.1632) ccw
  arc A56 (10.4462, -52.3625) -> (9.4415, -47.3835) centre (3.5497, -51.1632) ccw
  arc A57 (-9.1794, -48.0472) -> (-8.5127, -45.5527) centre (-13.5127, -45.5527) ccw
  arc A58 (-9.1794, -48.0472) -> (-8.9906, -50.8235) centre (-7.0127, -49.2944) ccw
  arc A59 (-8.0346, -52.946) -> (-8.9906, -50.8235) centre (-12.9463, -53.8816) ccw
  arc A60 (14.9651, -50.8235) -> (14.0092, -52.946) centre (18.9209, -53.8816) ccw
  arc A61 (14.9651, -50.8235) -> (15.1539, -48.0472) centre (12.9873, -49.2944) ccw
  arc A62 (14.4873, -45.5527) -> (15.1539, -48.0472) centre (19.4873, -45.5527) ccw
  arc A63 (10.9873, -32.7585) -> (10.6956, -31.3597) centre (7.4873, -32.7585) ccw
  arc A64 (-4.7211, -31.3597) -> (-5.0127, -32.7585) centre (-1.5127, -32.7585) ccw
  arc A65 (10.4873, -28.821) -> (8.6429, -28.2852) centre (9.4873, -28.821) ccw
  line L41 (10.4873, -28.821) -> (10.4873, -30.3606)
  arc A66 (10.4873, -30.3606) -> (10.6956, -31.3597) centre (12.9873, -30.3606) ccw
  arc A67 (-2.6684, -28.2852) -> (-4.5127, -28.821) centre (-3.5127, -28.821) ccw
  arc A68 (-4.7211, -31.3597) -> (-4.5127, -30.3606) centre (-7.0127, -30.3606) ccw
  line L42 (-4.5127, -30.3606) -> (-4.5127, -28.821)
  circle A69 centre (10.9873, -12.7944) radius 1.5
  circle A70 centre (10.9873, 3.2056) radius 1.5
  circle A71 centre (-5.0127, -12.7944) radius 1.5
  circle A72 centre (-5.0127, 3.2056) radius 1.5
  dimension "d217" = 4
  dimension "d218" = 4
  measures "d217" diameter of A49
  measures "d218" diameter of A50
extrude "Extrusion3'" cut sketch "Skizze20" along normal blind 7 contours A49 | A50 | A53 | A54 sketch seen with x (1, 0, 0) y (0, 1, 0) z (0, 0, 1) at (2.9873, 0.2056, -6) bodies 8 in component "Component"
extrude "Extrusion2''''" cut sketch "Skizze20" along normal blind 7 contours A49 | A50 | A53 | A54 sketch seen with x (0.989831, -0.142249, 0) y (-0.142249, -0.989831, 0) z (0, 0, -1) at (-24.4554, -5.7072, 6) bodies 12 in component "Component''''"
extrude "Extrusion1'''''''" cut sketch "Skizze20" along normal blind 7 contours A49 | A50 | A53 | A54 sketch seen with x (-0.989831, 0.142249, 0) y (-0.142249, -0.989831, 0) z (0, 0, 1) at (-19.2084, -21.6149, -3) bodies 14 in component "Component''''''"
fillet "Abrundung1'''" radius 5 2 edges at (-43.1261, -31.7237, 1.5) (-42.8551, -31.4062, 1.5) on bodies 12 in component "Component''''"
fillet "Abrundung1''''" radius 5 2 edges at (-31.6943, -48.1637, 1.5) (-31.9653, -48.4812, 1.5) on bodies 14 in component "Component''''''"
fillet "Abrundung2" radius 5 4 edges at (-11.8244, 30.3194, 1.5) (-9.3906, 27.5951, 1.5) (9.3906, 27.5951, 1.5) (11.8244, 30.3194, 1.5) on bodies 8 in component "Component"
sketch "Skizze21" plane through (0, 0, 6) normal (0, 0, 1) x (-1, 0, 0)
  arc A0 (-8.9028, -28.5618) -> (-8.7602, -28.3217) centre (-13.129, -25.8898) ccw
  arc A1 (-8.6409, -28.1329) -> (-8.7602, -28.3217) centre (-7.0127, -29.2944) ccw
  arc A2 (-3.4505, -24.2944) -> (-7.6767, -26.6224) centre (-3.4505, -29.2944) ccw
  line L0 (-3.4505, -24.2944) -> (2.9873, -24.2944)
  line L1 (2.9873, -24.2944) -> (2.9873, -21.2944)
  line L2 (2.9873, -21.2944) -> (-2.0127, -21.2944)
  arc A3 (-2.0127, -18.2944) -> (-2.0127, -21.2944) centre (-2.0127, -19.7944) ccw
  line L3 (-2.0127, -18.2944) -> (2.9873, -18.2944)
  line L4 (2.9873, -18.2944) -> (2.9873, -15.2944)
  line L5 (2.9873, -15.2944) -> (-7.914, -15.2944)
  arc A4 (-7.914, -15.2944) -> (-12.1561, -17.6477) centre (-7.914, -20.2944) ccw
  line L6 (-12.1561, -17.6477) -> (-24.9738, -38.1918)
  arc A5 (-29.7754, -45.2053) -> (-24.9738, -38.1918) centre (-109.8151, 14.7418) ccw
  line L7 (-29.7754, -45.2053) -> (-46.6298, -67.7088)
  arc A6 (-56.5231, -74.7617) -> (-46.6298, -67.7088) centre (-62.6377, -55.7193) ccw
  arc A7 (-56.5231, -74.7617) -> (-58.4629, -76.7028) centre (-55.6059, -77.6181) ccw
  arc A8 (-62.3739, -81.9285) -> (-58.4629, -76.7028) centre (-67.9861, -73.6518) ccw
  arc A9 (-62.3739, -81.9285) -> (-63.6615, -83.9975) centre (-60.6902, -84.4115) ccw
  line L8 (-63.6615, -83.9975) -> (-65.1229, -94.488)
  arc A10 (-65.1229, -94.488) -> (-62.3195, -96.587) centre (-63.142, -94.7639) ccw
  line L9 (-62.3195, -96.587) -> (-52.663, -92.2303)
  arc A11 (-52.663, -92.2303) -> (-51.0398, -90.411) centre (-53.8968, -89.4957) ccw
  arc A12 (-47.1289, -85.1853) -> (-51.0398, -90.411) centre (-41.5166, -93.4619) ccw
  arc A13 (-47.1289, -85.1853) -> (-45.8135, -82.7784) centre (-48.8125, -82.7023) ccw
  arc A14 (-41.832, -71.3016) -> (-45.8135, -82.7784) centre (-25.8199, -83.2854) ccw
  line L10 (-41.832, -71.3016) -> (-24.9852, -48.7917)
  arc A15 (-19.6077, -42.2094) -> (-24.9852, -48.7917) centre (55.0754, -108.7108) ccw
  line L11 (-19.6077, -42.2094) -> (-15.1756, -37.232)
  arc A16 (-15.1756, -37.232) -> (-10.2553, -30.7009) centre (-52.5171, -3.9813) ccw
  circle A17 centre (-14.804, -30.2009) radius 1
  arc A18 (-59.0559, -85.2371) -> (-59.355, -83.1585) centre (-59.2055, -84.1978) ccw
  line L12 (-59.0559, -85.2371) -> (-60.5406, -85.4508)
  arc A19 (-60.8397, -83.3722) -> (-60.5406, -85.4508) centre (-60.6902, -84.4115) ccw
  line L13 (-60.8397, -83.3722) -> (-59.355, -83.1585)
  arc A20 (-59.4121, -87.3355) -> (-61.1788, -87.8235) centre (-60.1889, -87.9652) ccw
  arc A21 (-59.4121, -87.3355) -> (-57.0641, -89.0932) centre (-54.7514, -83.5569) ccw
  arc A22 (-57.0349, -90.9259) -> (-57.0641, -89.0932) centre (-57.4496, -90.016) ccw
  line L14 (-57.0349, -90.9259) -> (-60.2795, -92.4046)
  arc A23 (-61.6842, -91.3529) -> (-60.2795, -92.4046) centre (-60.6943, -91.4947) ccw
  line L15 (-61.6842, -91.3529) -> (-61.1788, -87.8235)
  arc A24 (-54.5666, -77.4685) -> (-56.6452, -77.7676) centre (-55.6059, -77.6181) ccw
  line L16 (-54.5666, -77.4685) -> (-54.353, -78.9532)
  arc A25 (-56.4316, -79.2523) -> (-54.353, -78.9532) centre (-55.3923, -79.1028) ccw
  line L17 (-56.4316, -79.2523) -> (-56.6452, -77.7676)
  circle A26 centre (-54.7514, -83.5569) radius 2.5
  circle A27 centre (-7.0127, -19.7944) radius 1
  arc A28 (-53.0711, -87.8615) -> (-55.1497, -88.1606) centre (-54.1104, -88.011) ccw
  line L18 (-53.0711, -87.8615) -> (-52.8575, -89.3462)
  arc A29 (-54.9361, -89.6453) -> (-52.8575, -89.3462) centre (-53.8968, -89.4957) ccw
  line L19 (-54.9361, -89.6453) -> (-55.1497, -88.1606)
  line L20 (-50.4468, -81.8767) -> (-48.9621, -81.663)
  arc A30 (-48.663, -83.7416) -> (-48.9621, -81.663) centre (-48.8125, -82.7023) ccw
  line L21 (-48.663, -83.7416) -> (-50.1477, -83.9553)
  arc A31 (-50.4468, -81.8767) -> (-50.1477, -83.9553) centre (-50.2972, -82.916) ccw
  circle A32 centre (-14.804, -30.2009) radius 1.5
  circle A33 centre (-7.0127, -19.7944) radius 1.5
  line L22 (-8.4851, -27.9011) -> (-7.6767, -26.6224)
  line L23 (-10.2553, -30.7009) -> (-8.9028, -28.5618)
  arc A34 (-8.6409, -28.1329) -> (-8.4851, -27.9011) centre (-12.7113, -25.2291) ccw
  dimension "d231" = 3
  dimension "d232" = 3
  constraint concentric A17 A32
  constraint concentric A27 A33
  measures "d231" diameter of A32
  measures "d232" diameter of A33
extrude "Extrusion2'''''" cut sketch "Skizze21" against normal blind 3 contours A32 | A33 sketch seen with x (-0.989831, 0.142249, 0) y (-0.142249, -0.989831, 0) z (0, 0, 1) at (-19.2084, -21.6149, -3) bodies 14 in component "Component''''''"
sketch "Skizze22" plane through (0, 0, 38) normal (0, 0, 1) x (-1, 0, 0)
  circle A0 centre (-7.0127, -19.7944) radius 1.5
  circle A1 centre (15.4873, 34.6994) radius 1.5
  circle A2 centre (-7.0127, 10.2056) radius 1.5
  circle A3 centre (10.9873, -60.7944) radius 1.5
  circle A4 centre (12.9873, -19.7944) radius 1.5
  circle A5 centre (-9.5127, 34.6994) radius 1.5
  circle A6 centre (12.9873, 10.2056) radius 1.5
  circle A7 centre (-5.0127, -60.7944) radius 1.5
  arc A8 (6.3232, -2.4947) -> (5.9873, -3.6041) centre (7.9873, -3.6041) ccw
  line L0 (6.3232, -2.4947) -> (9.6552, 2.5034)
  arc A9 (11.4873, 1.9487) -> (9.6552, 2.5034) centre (10.4873, 1.9487) ccw
  line L1 (11.4873, 1.9487) -> (11.4873, -11.5374)
  arc A10 (9.6552, -12.0921) -> (11.4873, -11.5374) centre (10.4873, -11.5374) ccw
  line L2 (9.6552, -12.0921) -> (6.3232, -7.0941)
  arc A11 (5.9873, -5.9847) -> (6.3232, -7.0941) centre (7.9873, -5.9847) ccw
  line L3 (5.9873, -5.9847) -> (5.9873, -3.6041)
  arc A12 (11.4873, -27.4832) -> (9.6456, -26.9433) centre (10.4873, -27.4832) ccw
  line L4 (11.4873, -27.4832) -> (11.4873, -41.5523)
  arc A13 (9.6429, -42.088) -> (11.4873, -41.5523) centre (10.4873, -41.5523) ccw
  line L5 (9.6429, -42.088) -> (6.345, -36.8907)
  arc A14 (6.0338, -35.8191) -> (6.345, -36.8907) centre (8.0338, -35.8191) ccw
  line L6 (6.0338, -35.8191) -> (6.0338, -33.1598)
  arc A15 (6.3504, -32.0799) -> (6.0338, -33.1598) centre (8.0338, -33.1598) ccw
  line L7 (6.3504, -32.0799) -> (9.6456, -26.9433)
  arc A16 (4.09, -38.9361) -> (3.2456, -38.4719) centre (3.2456, -39.4719) ccw
  line L8 (4.09, -38.9361) -> (8.7639, -46.3021)
  arc A17 (8.2961, -48.9577) -> (8.7639, -46.3021) centre (7.0752, -47.3737) ccw
  line L9 (8.2961, -48.9577) -> (6.5954, -50.2685)
  arc A18 (4.7379, -50.5804) -> (6.5954, -50.2685) centre (5.3745, -48.6845) ccw
  arc A19 (4.7379, -50.5804) -> (1.2391, -50.5796) centre (2.9873, -55.7944) ccw
  arc A20 (-0.6186, -50.2666) -> (1.2391, -50.5796) centre (0.6033, -48.6833) ccw
  line L10 (-0.6186, -50.2666) -> (-2.3095, -48.9617)
  arc A21 (-2.7709, -46.2984) -> (-2.3095, -48.9617) centre (-1.0876, -47.3784) ccw
  line L11 (-2.7709, -46.2984) -> (1.9547, -38.932)
  arc A22 (2.7964, -38.4719) -> (1.9547, -38.932) centre (2.7964, -39.4719) ccw
  line L12 (2.7964, -38.4719) -> (3.2456, -38.4719)
  arc A23 (-0.3486, -7.0941) -> (-0.0127, -5.9847) centre (-2.0127, -5.9847) ccw
  line L13 (-0.3486, -7.0941) -> (-3.6807, -12.0921)
  arc A24 (-5.5127, -11.5374) -> (-3.6807, -12.0921) centre (-4.5127, -11.5374) ccw
  line L14 (-5.5127, -11.5374) -> (-5.5127, 1.9487)
  arc A25 (-3.6807, 2.5034) -> (-5.5127, 1.9487) centre (-4.5127, 1.9487) ccw
  line L15 (-3.6807, 2.5034) -> (-0.3486, -2.4947)
  arc A26 (-0.0127, -3.6041) -> (-0.3486, -2.4947) centre (-2.0127, -3.6041) ccw
  line L16 (-0.0127, -3.6041) -> (-0.0127, -5.9847)
  line L17 (-5.5127, -41.6055) -> (-5.5127, -38.2764)
  line L18 (-5.5127, -38.2764) -> (-5.3945, -27.4204)
  arc A27 (-3.5502, -26.8955) -> (-5.3945, -27.4204) centre (-4.3946, -27.4313) ccw
  line L19 (-3.5502, -26.8955) -> (-0.2775, -32.0531)
  arc A28 (0.0338, -33.1247) -> (-0.2775, -32.0531) centre (-1.9662, -33.1247) ccw
  line L20 (0.0338, -33.1247) -> (0.0338, -35.784)
  arc A29 (-0.2829, -36.8639) -> (0.0338, -35.784) centre (-1.9662, -35.784) ccw
  line L21 (-0.2829, -36.8639) -> (-3.671, -42.1455)
  arc A30 (-5.5127, -41.6055) -> (-3.671, -42.1455) centre (-4.5127, -41.6055) ccw
  circle A31 centre (2.9873, -55.7944) radius 3.5
  arc A32 (-2.9015, -51.2496) -> (-4.4977, -52.2126) centre (-3.5125, -52.0412) ccw
  line L22 (-2.9015, -51.2496) -> (-2.0972, -51.8703)
  arc A33 (-1.832, -53.1439) -> (-2.0972, -51.8703) centre (-2.7082, -52.662) ccw
  arc A34 (-1.832, -53.1439) -> (-2.2515, -54.1195) centre (2.9873, -55.7944) ccw
  arc A35 (-4.1892, -53.9863) -> (-2.2515, -54.1195) centre (-3.204, -53.815) ccw
  line L23 (-4.1892, -53.9863) -> (-4.4977, -52.2126)
  line L24 (1.3232, 0.4059) -> (-3.7366, 7.9956)
  arc A36 (-2.9071, 9.5503) -> (-3.7366, 7.9956) centre (-2.9045, 8.5503) ccw
  line L25 (-2.9071, 9.5503) -> (8.8963, 9.5799)
  arc A37 (9.7309, 8.0252) -> (8.8963, 9.5799) centre (8.8989, 8.5799) ccw
  line L26 (9.7309, 8.0252) -> (4.6514, 0.4059)
  arc A38 (1.3232, 0.4059) -> (4.6514, 0.4059) centre (2.9873, 1.5153) ccw
  line L27 (8.0742, -51.8736) -> (8.8754, -51.2561)
  arc A39 (10.4711, -52.2195) -> (8.8754, -51.2561) centre (9.4858, -52.0481) ccw
  line L28 (10.4711, -52.2195) -> (10.1638, -53.9863)
  arc A40 (8.2261, -54.1195) -> (10.1638, -53.9863) centre (9.1786, -53.815) ccw
  arc A41 (8.2261, -54.1195) -> (7.8082, -53.147) centre (2.9873, -55.7944) ccw
  arc A42 (8.0742, -51.8736) -> (7.8082, -53.147) centre (8.6847, -52.6656) ccw
  line L29 (8.7034, -22.8559) -> (4.1128, -30.0119)
  arc A43 (3.2711, -30.4719) -> (4.1128, -30.0119) centre (3.2711, -29.4719) ccw
  line L30 (3.2711, -30.4719) -> (2.8219, -30.4719)
  arc A44 (1.9776, -30.0077) -> (2.8219, -30.4719) centre (2.8219, -29.4719) ccw
  line L31 (1.9776, -30.0077) -> (-2.7352, -22.5805)
  arc A45 (-3.513, -19.8385) -> (-2.7352, -22.5805) centre (1.4866, -19.9016) ccw
  arc A46 (-3.513, -19.8385) -> (-3.5347, -19.4025) centre (-7.0127, -19.7944) ccw
  arc A47 (-2.7264, -16.0691) -> (-3.5347, -19.4025) centre (1.4338, -18.8426) ccw
  line L32 (-2.7264, -16.0691) -> (1.3232, -9.9947)
  arc A48 (4.6514, -9.9947) -> (1.3232, -9.9947) centre (2.9873, -11.1041) ccw
  line L33 (4.6514, -9.9947) -> (8.701, -16.0691)
  arc A49 (9.5093, -19.4025) -> (8.701, -16.0691) centre (4.5407, -18.8426) ccw
  arc A50 (9.5093, -19.4025) -> (9.4904, -19.9433) centre (12.9873, -19.7944) ccw
  arc A51 (8.7034, -22.8559) -> (9.4904, -19.9433) centre (4.495, -20.1561) ccw
  arc A52 (8.5923, -63.3467) -> (14.0385, -59.0797) centre (10.9873, -60.7944) ccw
  arc A53 (13.4856, -55.6946) -> (14.0385, -59.0797) centre (18.3973, -56.6301) ccw
  line L34 (13.4856, -55.6946) -> (14.9873, -47.811)
  line L35 (14.9873, -47.811) -> (14.9873, -24.6162)
  arc A54 (15.8696, -21.7798) -> (14.9873, -24.6162) centre (19.9873, -24.6162) ccw
  arc A55 (15.8696, -21.7798) -> (15.8696, -17.8089) centre (12.9873, -19.7944) ccw
  arc A56 (14.9873, -14.9726) -> (15.8696, -17.8089) centre (19.9873, -14.9726) ccw
  line L36 (14.9873, -14.9726) -> (14.9873, 3.6747)
  arc A57 (16.4873, 8.9425) -> (14.9873, 3.6747) centre (24.9873, 3.6747) ccw
  arc A58 (16.4873, 8.9425) -> (17.9873, 14.2103) centre (7.9873, 14.2103) ccw
  line L37 (17.9873, 14.2103) -> (17.9873, 30.6994)
  arc A59 (18.5755, 33.0523) -> (17.9873, 30.6994) centre (22.9873, 30.6994) ccw
  arc A60 (18.5755, 33.0523) -> (12.399, 33.0523) centre (15.4873, 34.6994) ccw
  arc A61 (12.9873, 30.6994) -> (12.399, 33.0523) centre (7.9873, 30.6994) ccw
  line L38 (12.9873, 30.6994) -> (12.9873, 19.4399)
  arc A62 (12.4033, 18.0275) -> (12.9873, 19.4399) centre (10.9873, 19.4399) ccw
  line L39 (12.4033, 18.0275) -> (9.5713, 15.1884)
  arc A63 (8.1603, 14.6008) -> (9.5713, 15.1884) centre (8.1553, 16.6008) ccw
  line L40 (8.1603, 14.6008) -> (-2.1828, 14.5748)
  arc A64 (-3.6003, 15.1588) -> (-2.1828, 14.5748) centre (-2.1879, 16.5748) ccw
  line L41 (-3.6003, 15.1588) -> (-6.4252, 17.9766)
  arc A65 (-7.0127, 19.3926) -> (-6.4252, 17.9766) centre (-5.0127, 19.3926) ccw
  line L42 (-7.0127, 19.3926) -> (-7.0127, 30.6994)
  arc A66 (-6.4245, 33.0523) -> (-7.0127, 30.6994) centre (-2.0127, 30.6994) ccw
  arc A67 (-6.4245, 33.0523) -> (-12.601, 33.0523) centre (-9.5127, 34.6994) ccw
  arc A68 (-12.0127, 30.6994) -> (-12.601, 33.0523) centre (-17.0127, 30.6994) ccw
  line L43 (-12.0127, 30.6994) -> (-12.0127, 14.2103)
  arc A69 (-12.0127, 14.2103) -> (-10.5127, 8.9425) centre (-2.0127, 14.2103) ccw
  arc A70 (-9.0127, 3.6747) -> (-10.5127, 8.9425) centre (-19.0127, 3.6747) ccw
  line L44 (-9.0127, 3.6747) -> (-9.0127, -14.9726)
  arc A71 (-9.8951, -17.8089) -> (-9.0127, -14.9726) centre (-14.0127, -14.9726) ccw
  arc A72 (-9.8951, -17.8089) -> (-9.8951, -21.7798) centre (-7.0127, -19.7944) ccw
  arc A73 (-9.0127, -24.6162) -> (-9.8951, -21.7798) centre (-14.0127, -24.6162) ccw
  line L45 (-9.0127, -24.6162) -> (-9.0127, -47.811)
  line L46 (-9.0127, -47.811) -> (-7.5111, -55.6946)
  arc A74 (-8.0639, -59.0797) -> (-7.5111, -55.6946) centre (-12.4228, -56.6301) ccw
  arc A75 (-8.0639, -59.0797) -> (-2.616, -63.345) centre (-5.0127, -60.7944) ccw
  arc A76 (-0.3989, -62.1366) -> (-2.616, -63.345) centre (0.8079, -66.9888) ccw
  line L47 (-0.3989, -62.1366) -> (0.5693, -61.8958)
  arc A77 (5.4047, -61.8978) -> (0.5693, -61.8958) centre (2.983, -71.6001) ccw
  line L48 (5.4047, -61.8978) -> (6.3819, -62.1417)
  arc A78 (8.5923, -63.3467) -> (6.3819, -62.1417) centre (5.171, -66.9929) ccw